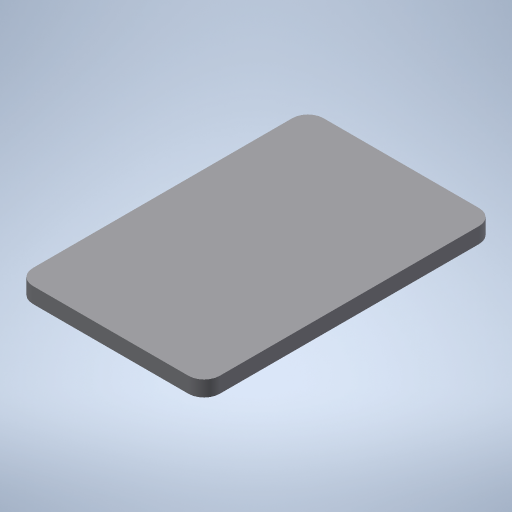
# Autodesk Inventor part: tapa caja servos
Saved by Autodesk Inventor 2023 (Build 270158000, 158)
## iProperties
Created: 2022-10-27
Part Number: tapa caja servos
Material: Generic
Document SubType Name: Modeling
Designer: Xiaba
Density: 1 g/cm^3
Appearance: Default
Author: Xiaba
Autodesk Inventor part; units mm, degrees
ref_plane "YZ Plane" through (0, 0, 0) normal (1, 0, 0) x (0, 1, 0)
ref_plane "XZ Plane" through (0, 0, 0) normal (0, 1, 0) x (-1, 0, 0)
ref_plane "XY Plane" through (0, 0, 0) normal (0, 0, 1) x (1, 0, 0)
sketch "Sketch1" plane through (0, 0, 0) normal (0, 1, 0) x (-1, 0, 0)
  line L0 (3, 0) -> (33, 0)
  line L1 (36, -3) -> (36, -53)
  line L2 (33, -56) -> (3, -56)
  line L3 (0, -53) -> (0, -3)
  arc A0 (33, -56) -> (36, -53) centre (33, -53) ccw
  arc A1 (0, -53) -> (3, -56) centre (3, -53) ccw
  arc A2 (3, 0) -> (0, -3) centre (3, -3) ccw
  arc A3 (36, -3) -> (33, 0) centre (33, -3) ccw
  point P0 (0, 0)
  point P1 (36, -56)
  point P2 (36, 0)
  point P3 (0, -56)
  dimension "d0" = 36
  dimension "d1" = 56
  dimension "d2" = 3
  constraints: 8 end point, 8 point on circle, 8 point on line, 8 tangent, 4 centre point, 3 equal radius, 2 parallel, 1 horizontal, 1 perpendicular
  measures "d0" distance of point (36, -56) point (0, -56)
  measures "d1" distance of point (36, 0) point (36, -56)
  measures "d2" radius of A0
extrude "Extrusion1" add sketch "Sketch1" along normal blind 3
body "Solid1"
